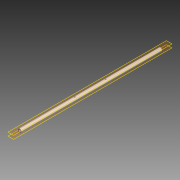
# Autodesk Inventor part: Zwischenstange
Saved by Autodesk Inventor 2013 (Build 170138000, 138)
## iProperties
Created: 2012-10-19
Part Number: Zwischenstange
Material: Aluminium
Document SubType Name: Modeling
Designer: fivef
Density: 1 g/cm^3
Author: fivef
Autodesk Inventor part; units mm, degrees
ref_plane "YZ Plane" through (0, 0, 0) normal (1, 0, 0) x (0, 1, 0)
ref_plane "XZ Plane" through (0, 0, 0) normal (0, 1, 0) x (-1, 0, 0)
ref_plane "XY Plane" through (0, 0, 0) normal (0, 0, 1) x (1, 0, 0)
sketch "Skizze1" plane through (0, 0, 0) normal (0, 1, 0) x (-1, 0, 0)
  circle A0 centre (0, 0) radius 5
  circle A1 centre (0, 0) radius 3
  dimension "d0" = 2
  dimension "d2" = 10
  dimension "d20" = 6
  constraints: 2 centre point, 2 coincident
  measures "d0" radial gap between concentric circles of A0 A1
  measures "d2" diameter of A0
  measures "d20" diameter of A1
extrude "Extrusion1" add sketch "Skizze1" along normal mid plane 410
ref_plane "Arbeitsebene2" through (0, 0, -5) normal (0, 0, 1) x (1, 0, 0)
ref_plane "Arbeitsebene1" through (-8, 108.509, 24.4581) normal (0, 0, 1) x (0, -1, 0)
sketch "Skizze3" plane through (0, 0, -5) normal (0, 0, 1) x (1, 0, 0)
  line L0 (0, 0) -> (0, 160.2649) construction
  point P0 (0, 0)
  point P1 (0, 80.1325)
  point P2 (0, 45)
  point P3 (0, -45)
  dimension "d8" = 45
  dimension "d10" = 45
  constraints: 2 coincident, 2 end point, 1 midpoint, 1 vertical
  measures "d8" distance of point (0, 45) point (0, 0)
  measures "d10" distance of point (0, -45) point (0, 0)
hole "Bohrung1" at (0, 45, -5) at (0, -45, -5) direction (0, 0, 1) diameter 4 end through all
ref_plane "Arbeitsebene4" through (0, 0, 5) normal (0, 0, 1) x (1, 0, 0)
thread "Gewinde1" size "M7x1" class "6H" standard "ANSI Metric M Profile" length 10
thread "Gewinde2" size "M7x1" class "6H" standard "ANSI Metric M Profile" length 10
